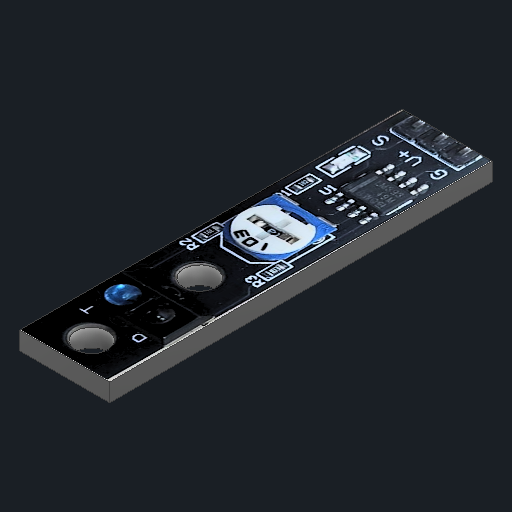
# Autodesk Inventor part: sensorInferior
Saved by Autodesk Inventor 2027 (Build 310192000, 192)
## iProperties
Created: 2025-06-04
Part Number: sensorInferior
Material: Generic
Document SubType Name: Modeling
Designer: cdavi
Density: 1 g/cm^3
Appearance: Default
Mass: 0.829642 g
Surface Area: 10.6226 cm^2
Volume: 0.829642 cm^3
Finish1_Area: 614,642 mm^2
Finish1_Appearance: Smooth - Black
Author: cdavi
Autodesk Inventor part; units mm, degrees
ref_plane "YZ Plane" through (0, 0, 0) normal (1, 0, 0) x (0, 1, 0)
ref_plane "XZ Plane" through (0, 0, 0) normal (0, 1, 0) x (-1, 0, 0)
ref_plane "XY Plane" through (0, 0, 0) normal (0, 0, 1) x (1, 0, 0)
sketch "Sketch1" plane through (0, 0, 0) normal (0, 1, 0) x (-1, 0, 0)
  line L0 (-5, 21.25) -> (5, 21.25)
  line L1 (5, 21.25) -> (5, -21.25)
  line L2 (5, -21.25) -> (-5, -21.25)
  line L3 (-5, -21.25) -> (-5, 21.25)
  line L4 (-5, 21.25) -> (5, -21.25) construction
  line L5 (5, 21.25) -> (-5, -21.25) construction
  circle A0 centre (0, 6.25) radius 1.8
  circle A1 centre (0, 18.25) radius 1.8
  point P0 (0, 0)
  dimension "d0" = 42.5
  dimension "d1" = 10
  dimension "d4" = 15
  dimension "d5" = 3.6
  dimension "d27" = 3.6
  dimension "d28" = 3
  constraints: 12 end point, 2 centre point, 2 midpoint, 2 parallel, 1 horizontal, 1 perpendicular, 1 vertical alignment
  measures "d0" distance of L0.end L1.end
  measures "d1" distance of L1.end L2.end
  measures "d4" distance from line of L0 A0.centre
  measures "d5" diameter of A0
  measures "d27" diameter of A1
  measures "d28" distance from line of L0 A1.centre
extrude "Extrusion1" add sketch "Sketch1" along normal blind 2
sketch "Sketch2" plane through (0, 2, 0) normal (0, 1, 0) x (1, 0, 0)
  line L0 (-5.1166, 21.6617) -> (4.9098, 21.6617) construction
  line L1 (4.9098, 21.6617) -> (4.9098, -21.1785) construction
  line L2 (4.9098, -21.1785) -> (-5.1166, -21.1785) construction
  line L3 (-5.1166, -21.1785) -> (-5.1166, 21.6617) construction
  point P0 (0, 0)
  constraints: 1 vertical, 2 other
decal "Decal1"
body "Solid1"
